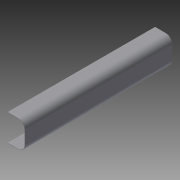
# Autodesk Inventor part: bumper_cloth
Saved by Autodesk Inventor 2015 SP1 (Build 190203100, 203)
## iProperties
Created: 2014-12-23
Part Number: bumper_cloth
Material: Generic
Document SubType Name: Modeling
Designer: Jarod
Density: 1 g/cm^3
Appearance: Default
Author: Jarod
Autodesk Inventor part; units mm, degrees
ref_plane "YZ Plane" through (0, 0, 0) normal (1, 0, 0) x (0, 1, 0)
ref_plane "XZ Plane" through (0, 0, 0) normal (0, 1, 0) x (-1, 0, 0)
ref_plane "XY Plane" through (0, 0, 0) normal (0, 0, 1) x (1, 0, 0)
sketch "Sketch1" plane through (0, 0, 0) normal (0, 0, 1) x (1, 0, 0)
  line L0 (0, 0) -> (19.05, 0) construction
  line L1 (19.05, 0) -> (19.05, 127) construction
  line L2 (19.05, 127) -> (0, 127) construction
  line L3 (0, 127) -> (0, 0) construction
  line L4 (19.05, 127) -> (82.55, 127) construction
  line L5 (82.55, 127) -> (82.55, 0) construction
  line L6 (82.55, 0) -> (19.05, 0) construction
  line L7 (19.05, 0) -> (19.05, 127) construction
  line L8 (0, 127) -> (50.8, 127)
  line L9 (50.8, 127) -> (50.8, 128.27)
  line L10 (50.8, 128.27) -> (0, 128.27)
  line L11 (0, 128.27) -> (0, 127)
  line L12 (0, 0) -> (50.8, 0)
  line L13 (50.8, 0) -> (50.8, -1.27)
  line L14 (50.8, -1.27) -> (0, -1.27)
  line L15 (0, -1.27) -> (0, 0)
  arc A0 (50.8, 0) -> (82.55, 31.75) centre (50.8, 31.75) ccw
  line L16 (50.8, 0) -> (82.55, 31.75) construction
  line L17 (50.8, 0) -> (95.7013, 0) construction
  arc A1 (82.55, 95.25) -> (50.8, 127) centre (50.8, 95.25) ccw
  line L18 (50.8, 127) -> (82.55, 95.25) construction
  line L19 (50.8, 127) -> (95.7013, 127) construction
  line L20 (82.55, 95.25) -> (83.82, 95.25)
  line L21 (83.82, 95.25) -> (83.82, 31.75)
  line L22 (83.82, 31.75) -> (82.55, 31.75)
  line L23 (82.55, 31.75) -> (82.55, 95.25)
  arc A2 (83.82, 95.25) -> (50.8, 128.27) centre (50.8, 95.25) ccw
  arc A3 (50.8, -1.27) -> (83.82, 31.75) centre (50.8, 31.75) ccw
  line L24 (82.55, 31.75) -> (83.82, 31.75)
  dimension "d0" = 19.05
  dimension "d1" = 127
  dimension "d2" = 63.5
  dimension "d3" = 127
  dimension "d4" = 50.8
  dimension "d5" = 1.27
  dimension "d6" = 50.8
  dimension "d7" = 1.27
  dimension "d8" = 45
  dimension "d9" = 31.75
  dimension "d10" = 45
  dimension "d11" = 31.75
  dimension "d12" = 1.27
  dimension "d13" = 63.5
  dimension "d14" = 33.02
  dimension "d15" = 33.02
  constraints: 50 end point, 10 parallel, 8 point on circle, 7 horizontal, 5 perpendicular, 4 centre point, 2 equal length, 2 point on line
  measures "d0" distance of L2.end L1.end
  measures "d1" distance of L1.end L0.end
  measures "d2" distance of L5.end L6.end
  measures "d3" distance of L4.end L5.end
  measures "d4" distance of L10.end L9.end
  measures "d5" distance of L9.end L8.end
  measures "d6" distance of L13.end L14.end
  measures "d7" distance of L12.end L13.end
  measures "d8" angle of L17 L16
  measures "d9" radius of A0
  measures "d10" angle of L18 L19
  measures "d11" radius of A1
  measures "d12" distance of L21.end L22.end
  measures "d13" distance of L20.end L21.end
  measures "d14" radius of A2
  measures "d15" radius of A3
extrude "Extrusion1" add sketch "Sketch1" along normal blind 711.2
sketch "Sketch2" plane through (0, 0, 711.2) normal (0, 0, 1) x (1, 0, 0)
  line L0 (50.8, 128.27) -> (0, 128.27) projected
  line L1 (0, 128.27) -> (0, 127) projected
  line L2 (0, 127) -> (50.8, 127) projected
  arc A0 (82.55, 95.25) -> (50.8, 127) centre (50.8, 95.25) ccw projected
  line L3 (82.55, 95.25) -> (82.55, 31.75) projected
  arc A1 (50.8, 0) -> (82.55, 31.75) centre (50.8, 31.75) ccw projected
  line L4 (50.8, 0) -> (0, 0) projected
  line L5 (0, 0) -> (0, -1.27) projected
  line L6 (0, -1.27) -> (50.8, -1.27) projected
  arc A2 (50.8, -1.27) -> (83.82, 31.75) centre (50.8, 31.75) ccw projected
  line L7 (83.82, 31.75) -> (83.82, 95.25) projected
  arc A3 (83.82, 95.25) -> (50.8, 128.27) centre (50.8, 95.25) ccw projected
  line L8 (0, 128.27) -> (-1.27, 128.27)
  line L9 (-1.27, 128.27) -> (-1.27, 102.87)
  line L10 (-1.27, 102.87) -> (0, 102.87)
  line L11 (0, 102.87) -> (0, 128.27)
  line L12 (0, -1.27) -> (-1.27, -1.27)
  line L13 (-1.27, -1.27) -> (-1.27, 24.13)
  line L14 (-1.27, 24.13) -> (0, 24.13)
  line L15 (0, 24.13) -> (0, -1.27)
  dimension "d18" = 1.27
  dimension "d19" = 25.4
  dimension "d20" = 1.27
  dimension "d21" = 25.4
  constraints: 16 end point, 4 parallel, 2 horizontal, 2 perpendicular
  measures "d18" distance of L10.end L9.end
  measures "d19" distance of L9.end L8.end
  measures "d20" distance of L13.end L14.end
  measures "d21" distance of L12.end L13.end
extrude "Extrusion2" add sketch "Sketch2" against normal blind 711.2 contours L1 L11 L10 L9 L8 | L12 L13 L14 L15 L5
body "Solid1"
